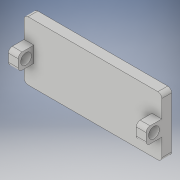
# Autodesk Inventor part: Pied
Saved by Autodesk Inventor 2019 (Build 230136000, 136)
## iProperties
Created: 2020-01-16
Part Number: Pied
Material: Générique
Document SubType Name: Modeling
Designer: Quentin
Density: 1 g/cm^3
Appearance: Par défaut
Author: Quentin
Autodesk Inventor part; units mm, degrees
ref_plane "YZ Plane" through (0, 0, 0) normal (1, 0, 0) x (0, 1, 0)
ref_plane "XZ Plane" through (0, 0, 0) normal (0, 1, 0) x (-1, 0, 0)
ref_plane "XY Plane" through (0, 0, 0) normal (0, 0, 1) x (1, 0, 0)
sketch "Esquisse1" plane through (0, 0, 0) normal (0, 0, 1) x (1, 0, 0)
  line L0 (2, 0) -> (68, 0)
  line L1 (70, 2) -> (70, 28)
  line L2 (68, 30) -> (2, 30)
  line L3 (0, 28) -> (0, 2)
  arc A0 (2, 30) -> (0, 28) centre (2, 28) ccw
  arc A1 (70, 28) -> (68, 30) centre (68, 28) ccw
  arc A2 (68, 0) -> (70, 2) centre (68, 2) ccw
  arc A3 (0, 2) -> (2, 0) centre (2, 2) ccw
  point P0 (0, 0)
  point P1 (70, 30)
  point P2 (70, 0)
  point P3 (0, 30)
  dimension "d0" = 70
  dimension "d1" = 30
  dimension "d14" = 2
  constraints: 8 end point, 8 point on circle, 8 point on line, 8 tangent, 4 centre point, 3 equal radius, 2 parallel, 1 horizontal, 1 perpendicular
  measures "d0" distance of point (0, 30) point (70, 30)
  measures "d1" distance of point (70, 0) point (70, 30)
  measures "d14" radius of A0
extrude "Extrusion1" add sketch "Esquisse1" along normal blind 5
sketch "Esquisse2" plane through (0, 0, 0) normal (-1, 0, 0) x (0, 0, 1)
  line L0 (5, 2) -> (5, 28) projected
  line L1 (5, 15) -> (5, 19)
  line L2 (5, 15) -> (5, 11)
  line L3 (5, 19) -> (11, 19)
  line L4 (13, 17) -> (13, 13)
  line L5 (11, 11) -> (5, 11)
  arc A0 (13, 17) -> (11, 19) centre (11, 17) ccw
  arc A1 (11, 11) -> (13, 13) centre (11, 13) ccw
  line L6 (5, 19) -> (12.4142, 11.5858) construction
  line L7 (5, 11) -> (12.4142, 18.4142) construction
  circle A2 centre (9, 15) radius 2.75
  line L8 (0, 2) -> (0, 28) projected
  line L9 (5, 2) -> (5, 28) projected
  line L10 (0, 2) -> (5, 2) projected
  line L11 (5, 28) -> (5, 2) projected
  line L12 (0, 28) -> (5, 28) projected
  line L13 (0, 2) -> (0, 28) projected
  line L14 (0, 2) -> (5, 2) projected
  line L15 (5, 28) -> (5, 2) projected
  line L16 (0, 28) -> (5, 28) projected
  line L17 (0, 2) -> (0, 28) projected
  line L18 (0, 28) -> (5, 28) projected
  line L19 (0, 2) -> (5, 2) projected
  point P0 (5, 0)
  point P1 (5, 30)
  point P2 (13, 19)
  dimension "d4" = 4
  dimension "d5" = 4
  dimension "d6" = 8
  dimension "d7" = 2
  dimension "d8" = 5.5
  constraints: 14 end point, 6 point on circle, 6 point on line, 4 tangent, 3 centre point, 2 perpendicular, 1 equal radius, 1 horizontal, 1 midpoint
  measures "d4" distance of L1.start L1.end
  measures "d5" distance of L1.start L2.end
  measures "d6" distance of L1.end point (13, 19)
  measures "d7" radius of A0
  measures "d8" diameter of A2
extrude "Extrusion2" add sketch "Esquisse2" against normal blind 5 contours L0 L3 A0 L4 A1 L5
sketch "Esquisse3" plane through (70, 0, 0) normal (1, 0, 0) x (0, 0, -1)
  line L0 (-11, 19) -> (-5, 19) projected
  line L1 (-5, 19) -> (-11, 19)
  line L2 (-11, 19) -> (-11, 19)
  line L3 (-13, 13) -> (-13, 17) projected
  line L4 (-13, 17) -> (-13, 13)
  line L5 (-11, 11) -> (-5, 11)
  line L6 (-5, 2) -> (-5, 28) projected
  line L7 (-5, 19) -> (-5, 11)
  arc A0 (-11, 19) -> (-13, 17) centre (-11, 17) ccw
  arc A1 (-13, 13) -> (-11, 11) centre (-11, 13) ccw
  circle A2 centre (-9, 15) radius 2.75 projected
  circle A3 centre (-9, 15) radius 2.5
  point P0 (0, 0)
  point P1 (-13, 19)
  point P2 (-5, 0)
  point P3 (-5, 30)
  dimension "d11" = 2
  constraints: 10 end point, 4 perpendicular, 4 point on circle, 4 point on line, 4 tangent, 3 centre point, 1 coincident, 1 equal radius, 1 horizontal
  measures "d11" radius of A0
extrude "Extrusion3" add sketch "Esquisse3" against normal blind 5 contours L0 L6 L5 A1 L3 A0
